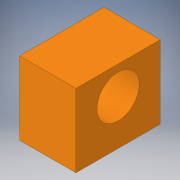
# Autodesk Inventor part: Hinge Block
Saved by Autodesk Inventor 2017 (Build 210142000, 142)
## iProperties
Created: 2017-01-12
Part Number: Hinge Block
Material: Generic
Document SubType Name: Modeling
Designer: Ben
Density: 1 g/cm^3
Appearance: Orange
Author: Ben
Autodesk Inventor part; units mm, degrees
ref_plane "YZ Plane" through (0, 0, 0) normal (1, 0, 0) x (0, 1, 0)
ref_plane "XZ Plane" through (0, 0, 0) normal (0, 1, 0) x (-1, 0, 0)
ref_plane "XY Plane" through (0, 0, 0) normal (0, 0, 1) x (1, 0, 0)
sketch "Sketch1" plane through (0, 0, 0) normal (1, 0, 0) x (0, 1, 0)
  circle A0 centre (0, 0) radius 4.7625
  line L0 (6.35, 9.525) -> (-10.16, 9.525)
  line L1 (-10.16, 9.525) -> (-10.16, -9.525)
  line L2 (-10.16, -9.525) -> (6.35, -9.525)
  line L3 (6.35, -9.525) -> (6.35, 9.525)
  line L4 (0, 0) -> (6.35, 0) construction
  dimension "d0" = 9.525
  dimension "d2" = 6.35
  dimension "d3" = 10.16
  dimension "d4" = 19.05
  constraints: 10 end point, 2 horizontal, 2 parallel, 1 centre point, 1 coincident, 1 midpoint, 1 perpendicular
  measures "d0" diameter of A0
  measures "d2" distance from line of point (0, 0) L3
  measures "d3" distance from line of point (0, 0) L1
  measures "d4" distance of L2.end L0.start
extrude "Extrusion1" add sketch "Sketch1" along normal blind 12.7
body "Solid1"
